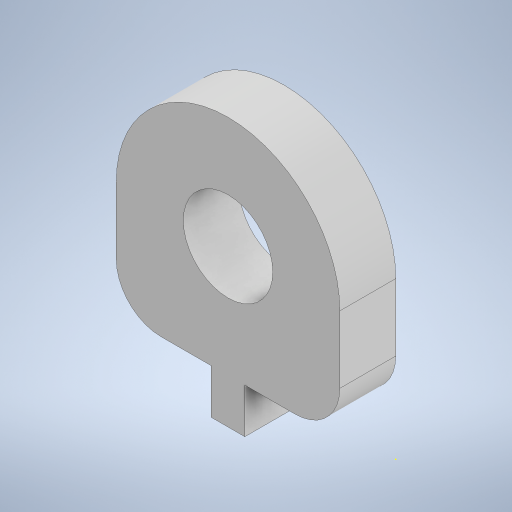
# Autodesk Inventor part: Knuckle Attachment DirectInsert
Saved by Autodesk Inventor 2023 (Build 270158000, 158)
## iProperties
Created: 2023-04-04
Part Number: Knuckle Attachment DirectInsert
Material: Generic
Document SubType Name: Modeling
Designer: 1senadi
Density: 1 g/cm^3
Appearance: Default
Author: 1senadi
Autodesk Inventor part; units mm, degrees
ref_plane "YZ Plane" through (0, 0, 0) normal (1, 0, 0) x (0, 1, 0)
ref_plane "XZ Plane" through (0, 0, 0) normal (0, 1, 0) x (-1, 0, 0)
ref_plane "XY Plane" through (0, 0, 0) normal (0, 0, 1) x (1, 0, 0)
sketch "Sketch1" plane through (0, 0, 0) normal (0, 1, 0) x (-1, 0, 0)
  line L0 (0, 0) -> (0, -2.5)
  line L1 (0, -2.5) -> (10, -2.5)
  line L2 (10, -2.5) -> (10, 0)
  line L3 (10, 0) -> (0, 0)
  dimension "d0" = 2.5
  dimension "d1" = 10
  dimension "d2" = 90
  dimension "d3" = 2.5
  constraints: 8 end point, 2 perpendicular, 1 vertical
  measures "d0" distance of L0.start L0.end
  measures "d1" distance of L0.end L1.end
  measures "d2" angle of L1 L0
  measures "d3" distance of L1.end L2.end
extrude "Extrusion1" add sketch "Sketch1" along normal blind 12
sketch "Sketch4" plane through (0, 0, -2.5) normal (0, 0, -1) x (-1, 0, 0)
  line L0 (0, 0) -> (0, 2)
  line L1 (0, 0) -> (0, 12) projected
  line L2 (0, 2) -> (4, 2)
  line L3 (10, 0) -> (10, 12) projected
  line L4 (4, 2) -> (0, 0)
  line L5 (0, 0) -> (10, 0) projected
  line L6 (10, 0) -> (10, 2)
  line L7 (10, 2) -> (6, 2)
  line L8 (6, 2) -> (10, 0)
  dimension "d9" = 2
  dimension "d10" = 4
  dimension "d11" = 2
  dimension "d12" = 4
  constraints: 12 end point, 2 perpendicular, 2 point on line
  measures "d9" distance of L0.start L0.end
  measures "d10" distance of L0.end L2.end
  measures "d11" distance of L3.start L6.end
  measures "d12" distance of L6.end L7.end
extrude "Extrusion3" cut sketch "Sketch4" against normal up to surface (2.5 mm away)
sketch "Sketch5" plane through (0, 12, -2.5) normal (0, 0, -1) x (-1, 0, 0)
  point P0 (0, -12)
sketch "Sketch6" plane through (0, 12, -2.5) normal (0, 0, -1) x (-1, 0, 0)
  line L0 (0, -10) -> (0, 0) projected
  line L1 (0, -5) -> (10, -5)
  line L2 (10, -10) -> (10, 0) projected
  line L3 (0, 0) -> (10, 0) projected
  line L4 (5, 0) -> (5, -10)
  circle A0 centre (5, -5) radius 2
  point P0 (0, -12)
  dimension "d15" = 4
  constraints: 4 end point, 4 midpoint, 1 centre point, 1 vertical
  measures "d15" diameter of A0
extrude "Extrusion4" cut sketch "Sketch6" against normal up to surface (2.5 mm away) contours A0 L4 L1 | L1 L4 A0 | L4 A0 L1 | L1 A0 L4
fillet "Fillet1" radius 2 4 edges at (0, 12, -1.25) (0, 2, -1.25) (-10, 12, -1.25) (-10, 2, -1.25)
fillet "Fillet2" radius 0.5 1 edges at (0, 0, -1.25)
fillet "Fillet3" radius 0.5 1 edges at (-10, 0, -1.25)
sketch "Sketch7" plane through (-8, 12, 0) normal (0, 0, 1) x (1, 0, 0)
  circle A0 centre (3, -5) radius 2 projected
  arc A1 (8, -2) -> (6, 0) centre (6, -2) ccw projected
  circle A2 centre (3, -5) radius 5
  line L0 (6, 0) -> (0, 0) projected
  arc A3 (-0.1056, -11.0528) -> (0.118, -12) centre (0.118, -11.5) ccw projected
  line L1 (0.118, -12) -> (5.882, -12) projected
  arc A4 (5.882, -12) -> (6.1056, -11.0528) centre (5.882, -11.5) ccw projected
  line L2 (6.1056, -11.0528) -> (4, -10) projected
  line L3 (4, -10) -> (6, -10) projected
  arc A5 (6, -10) -> (8, -8) centre (6, -8) ccw projected
  line L4 (8, -8) -> (8, -2) projected
  arc A6 (8, -2) -> (6, 0) centre (6, -2) ccw projected
  line L5 (0, 0) -> (6, 0) projected
  arc A7 (0, 0) -> (-2, -2) centre (0, -2) ccw projected
  line L6 (-2, -8) -> (-2, -2) projected
  arc A8 (-2, -8) -> (0, -10) centre (0, -8) ccw projected
  line L7 (0, -10) -> (2, -10) projected
  line L8 (2, -10) -> (-0.1056, -11.0528) projected
  circle A9 centre (3, -5) radius 2 projected
  point P0 (8, -12)
  point P1 (-2, -5)
  point P2 (3, 0)
  point P3 (8, -5)
  point P4 (8, -2)
  constraints: 1 centre point, 1 coincident, 1 tangent
extrude "Extrusion5" cut sketch "Sketch7" against normal up to surface (2.5 mm away) contours L4 A2 L0 A1 | A2 L6 A7 L0
sketch "Sketch8" plane through (-8, 2, 0) normal (0, 0, 1) x (1, 0, 0)
  circle A0 centre (3, 5) radius 2 projected
  arc A1 (8, 5) -> (-2, 5) centre (3, 5) ccw projected
  line L0 (-2, 2) -> (-2, 5) projected
  arc A2 (-2, 2) -> (0, 0) centre (0, 2) ccw projected
  line L1 (0, 0) -> (2, 0) projected
  line L2 (2, 0) -> (-0.1056, -1.0528) projected
  arc A3 (-0.1056, -1.0528) -> (0.118, -2) centre (0.118, -1.5) ccw projected
  line L3 (0.118, -2) -> (5.882, -2) projected
  arc A4 (5.882, -2) -> (6.1056, -1.0528) centre (5.882, -1.5) ccw projected
  line L4 (6.1056, -1.0528) -> (4, 0) projected
  line L5 (4, 0) -> (6, 0) projected
  arc A5 (6, 0) -> (8, 2) centre (6, 2) ccw projected
  line L6 (8, 2) -> (8, 5) projected
  line L7 (2, 0) -> (0, 0) projected
  line L8 (2, 0) -> (2, -2)
  line L9 (5.882, -2) -> (0.118, -2) projected
  line L10 (4, 0) -> (4, -2)
  line L11 (3, 0) -> (2.25, 0)
  line L12 (3, 0) -> (3.75, 0)
  line L13 (3.75, 0) -> (3.75, -2)
  line L14 (2.25, 0) -> (2.25, -2)
  line L15 (2.25, -2) -> (3.75, -2)
  line L16 (-0.1056, -1.0528) -> (2, 0) projected
  line L17 (2, 0) -> (4, 0)
  line L18 (2, -2) -> (4, -2)
  point P0 (8, -2)
  point P1 (2, -2)
  point P2 (2.25, 0)
  point P3 (2.25, -2)
  point P4 (3.75, 0)
  dimension "d25" = 0.75
  dimension "d26" = 0.75
  constraints: 18 end point, 4 perpendicular, 4 point on line, 2 collinear, 1 horizontal, 1 parallel
  measures "d25" distance of L11.start L11.end
  measures "d26" distance of L11.start L12.end
extrude "Extrusion6" cut sketch "Sketch8" against normal up to surface (2.5 mm away) contours L4 A4 L3 L10 | L10 L3 L13 L17 | L8 L3 A3 L2 | L17 L14 L3 L8
body "Solid1"
